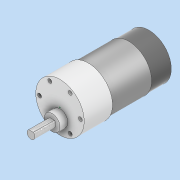
# Autodesk Inventor part: Motor
Saved by Autodesk Inventor 2021 (Build 250183000, 183)
## iProperties
Created: 2021-02-01
Part Number: Motor
Material: Generic
Document SubType Name: Modeling
Designer: garre
Density: 1 g/cm^3
Appearance: Default
Author: garre
Autodesk Inventor part; units mm, degrees
ref_plane "YZ Plane" through (0, 0, 0) normal (1, 0, 0) x (0, 1, 0)
ref_plane "XZ Plane" through (0, 0, 0) normal (0, 1, 0) x (-1, 0, 0)
ref_plane "XY Plane" through (0, 0, 0) normal (0, 0, 1) x (1, 0, 0)
sketch "Sketch1" plane through (0, 0, 0) normal (0, 0, 1) x (1, 0, 0)
  point P0 (0, 0)
sketch "Sketch2" plane through (0, 0, 0) normal (0, 0, 1) x (1, 0, 0)
  circle A0 centre (0, 0) radius 18.4
  dimension "d0" = 36.8
  constraints: 1 centre point, 1 coincident
  measures "d0" diameter of A0
extrude "Extrusion1" add sketch "Sketch2" against normal blind 21.5
sketch "Sketch3" plane through (0, 0, -21.5) normal (0, 0, -1) x (-1, 0, 0)
  circle A0 centre (0, 0) radius 17.4
  dimension "d3" = 34.8
  constraints: 1 centre point, 1 coincident
  measures "d3" diameter of A0
extrude "Extrusion2" add sketch "Sketch3" along normal blind 30.7
sketch "Sketch4" plane through (0, 0, -52.2) normal (0, 0, -1) x (-1, 0, 0)
  circle A0 centre (0, 0) radius 17
  dimension "d6" = 34
  constraints: 1 centre point, 1 coincident
  measures "d6" diameter of A0
extrude "Extrusion3" add sketch "Sketch4" along normal blind 15.4
sketch "Sketch5" plane through (0, 0, 0) normal (0, 0, 1) x (1, 0, 0)
  circle A0 centre (-15.5, 0) radius 1.5
  circle A1 centre (0, 0) radius 18.4 projected
  line L0 (-18.4, 0) -> (18.4, 0)
  line L1 (-1.5961, -18.3306) -> (-1.5961, -18.3306)
  line L2 (0, 18.4) -> (0, -18.4)
  circle A2 centre (0, -7) radius 6
  circle A3 centre (15.5, 0) radius 1.5
  circle A4 centre (0, 0) radius 15.5
  line L3 (-11.863, 20.6629) -> (9.25, -15.9059)
  circle A5 centre (0, 0) radius 18.4 projected
  line L4 (-9.2, -15.9349) -> (9.2, 15.9349)
  circle A6 centre (7.8, -13.3944) radius 1.5
  circle A7 centre (7.75, 13.4234) radius 1.5
  circle A8 centre (-7.75, -13.4234) radius 1.5
  circle A9 centre (-7.6999, 13.4522) radius 1.5
  point P0 (7.75, 13.4234)
  point P1 (7.8, -13.3944)
  dimension "d10" = 3
  dimension "d11" = 12
  dimension "d12" = 7
  dimension "d15" = 3
  dimension "d16" = 31
  dimension "d17" = 2.9
  dimension "d19" = 60
  dimension "d20" = 60
  dimension "d21" = 3
  dimension "d22" = 3
  dimension "d23" = 3
  dimension "d24" = 3
  constraints: 11 point on circle, 10 end point, 8 centre point, 6 point on line, 4 coincident, 3 midpoint, 1 horizontal, 1 tangent, 1 vertical, 4 other
  measures "d10" diameter of A0
  measures "d11" diameter of A2
  measures "d12" vertical distance of A2.centre A0.centre
  measures "d15" diameter of A3
  measures "d16" distance of A3.centre A0.centre
  measures "d17" distance of L0.start A0.centre
  measures "d19" angle of L0 L3
  measures "d20" angle of L0 L4
  measures "d21" diameter of A6
  measures "d22" diameter of A7
  measures "d23" diameter of A8
  measures "d24" diameter of A9
extrude "Extrusion4" add sketch "Sketch5" along normal blind 6 contours A2 L3 L2 | L2 A2 L4 | L4 A2 | A2 L3 picked at (-1.9225, -8.5027)
extrude "Extrusion5" cut sketch "Sketch5" against normal blind 3 contours L0 A4 A0 | A0 A4 L0 | A4 L0 A0 | A0 L0 A4 | A9 L3 A4 | A4 L3 A9 | A8 L4 A4 | A4 L4 A8 | L3 A9 A4 | A4 A9 L3 | L4 A8 A4 | A4 A8 L4 | A3 A4 L0 | L0 A4 A3 | A7 A4 L4 | L4 A4 A7 | A4 A3 L0 | L0 A3 A4 | A7 L4 A4 | L4 A7 A4 | A6 L3 A4 | A4 L3 A6 | L3 A4 A6 | A4 L3 A6
sketch "Sketch6" plane through (0, -7, 6) normal (0, 0, 1) x (1, 0, 0)
  circle A0 centre (0, 0) radius 6 projected
  circle A1 centre (0, 0) radius 3
  point P0 (0, 7)
  dimension "d27" = 6
  constraints: 1 centre point, 1 coincident
  measures "d27" diameter of A1
extrude "Extrusion6" add sketch "Sketch6" along normal blind 16 contours A1
sketch "Sketch7" plane through (0, -7, 22) normal (0, 0, 1) x (1, 0, 0)
  line L0 (-6, 3) -> (6, 3)
  line L1 (6, 3) -> (6, 2.4)
  line L2 (6, 2.4) -> (-6, 2.4)
  line L3 (-6, 2.4) -> (-6, 3)
  circle A0 centre (0, 0) radius 6 projected
  circle A1 centre (0, 0) radius 3 projected
  circle A2 centre (0, 0) radius 3 projected
  line L4 (0, 3) -> (0, -3)
  point P0 (0, 7)
  dimension "d30" = 0.6
  constraints: 10 end point, 2 midpoint, 2 parallel, 2 point on circle, 1 horizontal, 1 perpendicular, 1 vertical, 1 vertical alignment, 1 other
  measures "d30" distance of L2.end L0.start
extrude "Extrusion7" cut sketch "Sketch7" against normal up to surface (16 mm away) contours L0 A0 L2 L3 | L0 A1 L2 A0 | L0 A0 L2 A1 | L4 L2 A1 | A1 L2 L4 | L0 L1 L2 A0 picked at (-1.016, 2.5094) picked at (1.016, 2.5094)
body "Solid1"
